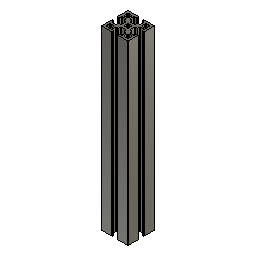
Extruder_MBXL_Cover v6 (Autodesk Fusion 360 archive; units mm, degrees)
design "MakerBeam XL"
Autodesk Fusion 360 part; units mm, degrees
sketch "Sketch1" plane through (0, 0, 0) normal (0, 0, 1) x (1, 0, 0)
  line L0 (-7.5, 7.5) -> (7.5, 7.5)
  line L1 (7.5, 7.5) -> (7.5, -7.5)
  line L2 (7.5, -7.5) -> (-7.5, -7.5)
  line L3 (-7.5, -7.5) -> (-7.5, 7.5)
  line L4 (-7.5, 7.5) -> (7.5, -7.5) construction
  line L5 (7.5, 7.5) -> (-7.5, -7.5) construction
  circle A0 centre (0, 0) radius 1.275
  line L6 (1.125, 1.125) -> (-1.125, 1.125)
  line L7 (-1.125, 1.125) -> (-1.125, -1.125)
  line L8 (-1.125, -1.125) -> (1.125, -1.125)
  line L9 (1.125, -1.125) -> (1.125, 1.125)
  line L10 (1.125, 1.125) -> (-1.125, -1.125) construction
  line L11 (-1.125, 1.125) -> (1.125, -1.125) construction
  circle A1 centre (5, 5) radius 1.275
  line L12 (6.125, 6.125) -> (3.875, 6.125)
  line L13 (3.875, 6.125) -> (3.875, 3.875)
  line L14 (3.875, 3.875) -> (6.125, 3.875)
  line L15 (6.125, 3.875) -> (6.125, 6.125)
  line L16 (6.125, 6.125) -> (3.875, 3.875) construction
  line L17 (3.875, 6.125) -> (6.125, 3.875) construction
  line L18 (7.5, 1.5) -> (2.5, 1.5)
  line L19 (2.5, 1.5) -> (2.5, -1.5)
  line L20 (2.5, -1.5) -> (7.5, -1.5)
  line L21 (7.5, -1.5) -> (7.5, 1.5)
  line L22 (7.5, 1.5) -> (2.5, -1.5) construction
  line L23 (2.5, 1.5) -> (7.5, -1.5) construction
  line L24 (6.4, 2.85) -> (3.9, 2.85)
  line L25 (3.9, 2.85) -> (3.9, -2.85)
  line L26 (3.9, -2.85) -> (6.4, -2.85)
  line L27 (6.4, -2.85) -> (6.4, 2.85)
  line L28 (6.4, 2.85) -> (3.9, -2.85) construction
  line L29 (3.9, 2.85) -> (6.4, -2.85) construction
  line L30 (-3.875, 3.875) -> (-3.875, 6.125)
  line L31 (-1.5, 7.5) -> (1.5, 2.5) construction
  line L32 (-1.5, 7.5) -> (-1.5, 2.5)
  line L33 (-6.125, 6.125) -> (-6.125, 3.875)
  line L34 (1.5, 2.5) -> (1.5, 7.5)
  line L35 (-6.125, 6.125) -> (-3.875, 3.875) construction
  circle A2 centre (-5, 5) radius 1.275
  line L36 (-1.5, 2.5) -> (1.5, 7.5) construction
  line L37 (-6.125, 3.875) -> (-3.875, 6.125) construction
  line L38 (-2.85, 6.4) -> (2.85, 3.9) construction
  line L39 (1.5, 7.5) -> (-1.5, 7.5)
  line L40 (-2.85, 3.9) -> (2.85, 3.9)
  line L41 (2.85, 3.9) -> (2.85, 6.4)
  line L42 (-6.125, 3.875) -> (-3.875, 3.875)
  line L43 (-2.85, 3.9) -> (2.85, 6.4) construction
  line L44 (-3.875, 6.125) -> (-6.125, 6.125)
  line L45 (-1.5, 2.5) -> (1.5, 2.5)
  line L46 (-2.85, 6.4) -> (-2.85, 3.9)
  line L47 (2.85, 6.4) -> (-2.85, 6.4)
  line L48 (-3.875, -3.875) -> (-6.125, -3.875)
  line L49 (-7.5, -1.5) -> (-2.5, 1.5) construction
  line L50 (-7.5, -1.5) -> (-2.5, -1.5)
  line L51 (-6.125, -6.125) -> (-3.875, -6.125)
  line L52 (-2.5, 1.5) -> (-7.5, 1.5)
  line L53 (-6.125, -6.125) -> (-3.875, -3.875) construction
  circle A3 centre (-5, -5) radius 1.275
  line L54 (-2.5, -1.5) -> (-7.5, 1.5) construction
  line L55 (-3.875, -6.125) -> (-6.125, -3.875) construction
  line L56 (-6.4, -2.85) -> (-3.9, 2.85) construction
  line L57 (-7.5, 1.5) -> (-7.5, -1.5)
  line L58 (-3.9, -2.85) -> (-3.9, 2.85)
  line L59 (-3.9, 2.85) -> (-6.4, 2.85)
  line L60 (-3.875, -6.125) -> (-3.875, -3.875)
  line L61 (-3.9, -2.85) -> (-6.4, 2.85) construction
  line L62 (-6.125, -3.875) -> (-6.125, -6.125)
  line L63 (-2.5, -1.5) -> (-2.5, 1.5)
  line L64 (-6.4, -2.85) -> (-3.9, -2.85)
  line L65 (-6.4, 2.85) -> (-6.4, -2.85)
  line L66 (3.875, -3.875) -> (3.875, -6.125)
  line L67 (1.5, -7.5) -> (-1.5, -2.5) construction
  line L68 (1.5, -7.5) -> (1.5, -2.5)
  line L69 (6.125, -6.125) -> (6.125, -3.875)
  line L70 (-1.5, -2.5) -> (-1.5, -7.5)
  line L71 (6.125, -6.125) -> (3.875, -3.875) construction
  circle A4 centre (5, -5) radius 1.275
  line L72 (1.5, -2.5) -> (-1.5, -7.5) construction
  line L73 (6.125, -3.875) -> (3.875, -6.125) construction
  line L74 (2.85, -6.4) -> (-2.85, -3.9) construction
  line L75 (-1.5, -7.5) -> (1.5, -7.5)
  line L76 (2.85, -3.9) -> (-2.85, -3.9)
  line L77 (-2.85, -3.9) -> (-2.85, -6.4)
  line L78 (6.125, -3.875) -> (3.875, -3.875)
  line L79 (2.85, -3.9) -> (-2.85, -6.4) construction
  line L80 (3.875, -6.125) -> (6.125, -6.125)
  line L81 (1.5, -2.5) -> (-1.5, -2.5)
  line L82 (2.85, -6.4) -> (2.85, -3.9)
  line L83 (-2.85, -6.4) -> (2.85, -6.4)
  point P0 (5, 5)
  point P1 (5, 0)
  point P2 (5.15, 0)
  point P3 (-5, 5)
  point P4 (0, 5)
  point P5 (0, 5.15)
  point P6 (-5, -5)
  point P7 (-5, 0)
  point P8 (-5.15, 0)
  point P9 (5, -5)
  point P10 (0, -5)
  point P11 (0, -5.15)
  dimension "d1" = 15
  dimension "d2" = 15
  dimension "d3" = 2.55
  dimension "d4" = 2.25
  dimension "d5" = 2.25
  dimension "d6" = 2.55
  dimension "d7" = 2.25
  dimension "d8" = 2.25
  dimension "d9" = 5
  dimension "d10" = 3
  dimension "d11" = 2.5
  dimension "d12" = 5.7
  dimension "d13" = 1.1
  dimension "d15" = 360
  constraint horizontal L0
  constraint perpendicular L0 L1
  constraint parallel L0 L2
  constraint parallel L1 L3
  constraint coincident L4 A0.centre
  constraint coincident L5 A0.centre
  constraint coincident A0.centre origin
  constraint horizontal L6
  constraint perpendicular L6 L7
  constraint parallel L6 L8
  constraint parallel L7 L9
  constraint coincident L10 A0.centre
  constraint coincident L11 A0.centre
  constraint coincident L5 P0
  constraint horizontal L12
  constraint perpendicular L12 L13
  constraint parallel L12 L14
  constraint parallel L13 L15
  constraint coincident L16 P0
  constraint coincident L17 P0
  constraint coincident P0 A1.centre
  constraint horizontal L18
  constraint perpendicular L18 L19
  constraint parallel L18 L20
  constraint parallel L19 L21
  constraint coincident L22 P1
  constraint coincident L23 P1
  constraint horizontal L24
  constraint perpendicular L24 L25
  constraint parallel L24 L26
  constraint parallel L25 L27
  constraint coincident L28 P2
  constraint coincident L29 P2
  measures "d1" distance of L1.end L2.end
  measures "d2" distance of L0.end L1.end
  measures "d3" diameter of A0
  measures "d4" distance of L7.end L8.end
  measures "d5" distance of L6.end L7.end
  measures "d6" diameter of A1
  measures "d7" distance of L13.end L14.end
  measures "d8" distance of L12.end L13.end
  measures "d9" distance of L19.end L20.end
  measures "d10" distance of L18.end L19.end
  measures "d11" distance of L25.end L26.end
  measures "d12" distance of L24.end L25.end
  measures "d13" distance of L1 L27
extrude "Extrude1" add sketch "Sketch1" against normal blind 100 contours L0 L1 L2 L3 L18 L19 L20 L24 L25 L26 L27 L32 L34 L40 L41 L45 L46 L47 L50 L52 L58 L59 L63 L64 L65 L68 L70 L76 L77 L81 L82 L83
fillet "Fillet1" radius 0.25 112 edges at (-7.5, 7.5, -50) (3.875, 3.875, -50) (3.875, -4.4, -50) (1.5, 3.9, -50) (1.125, 0.6, -50) (1.5, -6.4, -50) (1.5, -3.9, -50) (-3.9, 2.85, -50) (-6.125, 3.875, -50) (-6.4, 1.5, -50) (-6.125, 6.125, -50) (-2.5, 1.5, -50) (-1.5, 2.5, -50) (3.875, -6.125, -50) (-1.5, -3.9, -50) (-3.875, -4.4, -50) (6.125, -4.4, -50) (-2.85, 6.4, -50) (-6.125, -3.875, -50) (2.85, -6.4, -50) (7.5, -7.5, -50) (-2.85, 3.9, -50) (-2.5, -1.5, -50) (0.6, 1.125, -50) (6.4, 2.85, -50) (1.125, -1.125, -50) (7.5, -1.5, -50) (6.125, -6.125, -50) (-3.875, -5.6, -50) (0.6, -1.125, -50) (-6.125, 4.4, -50) (5.6, -6.125, -50) (3.9, -2.85, -50) (3.9, 1.5, -50) (5.6, 6.125, -50) (-3.9, -1.5, -50) (-3.875, 5.6, -50) (1.5, 7.5, -50) (5.6, 3.875, -50) (-5.6, 3.875, -50) (-4.4, -6.125, -50) (-0.6, -1.125, -50) (3.875, 4.4, -50) (6.125, -3.875, -50) (1.5, -2.5, -50) (6.125, 6.125, -50) (-1.5, -6.4, -50) (-6.4, -2.85, -50) (2.85, -3.9, -50) (4.4, 3.875, -50) (-4.4, 3.875, -50) (1.5, -7.5, -50) (-5.6, -3.875, -50) (-1.125, -1.125, -50) (7.5, 7.5, -50) (-3.875, 4.4, -50) (-4.4, 6.125, -50) (-6.125, -4.4, -50) (2.5, 1.5, -50) (-5.6, 6.125, -50) (6.4, 1.5, -50) (1.5, 6.4, -50) (1.125, -0.6, -50) (2.85, 3.9, -50) (-6.125, -6.125, -50) (4.4, -6.125, -50) (-1.125, -0.6, -50) (1.125, 1.125, -50) (-6.4, -1.5, -50) (-7.5, -7.5, -50) (6.125, -5.6, -50) (6.125, 3.875, -50) (-1.5, 7.5, -50) (3.875, 5.6, -50) (3.9, -1.5, -50) (-1.125, 0.6, -50) (-3.9, -2.85, -50) (-3.875, 6.125, -50) (2.85, 6.4, -50) (3.9, 2.85, -50) (-1.5, 6.4, -50) (-3.875, 3.875, -50) (3.875, -5.6, -50) (-2.85, -6.4, -50) (-1.5, 3.9, -50) (3.875, -3.875, -50) (-3.875, -6.125, -50) (-6.4, 2.85, -50) (3.875, 6.125, -50) (-5.6, -6.125, -50) (-7.5, -1.5, -50) (-3.9, 1.5, -50) (-0.6, 1.125, -50) (1.5, 2.5, -50) (6.125, 4.4, -50) (-4.4, -3.875, -50) (-1.5, -2.5, -50) (-3.875, -3.875, -50) (4.4, -3.875, -50) (5.6, -3.875, -50) (4.4, 6.125, -50) (6.4, -1.5, -50) (2.5, -1.5, -50) (-6.125, -5.6, -50) (-1.125, 1.125, -50) (-7.5, 1.5, -50) (-2.85, -3.9, -50) (7.5, 1.5, -50) (6.125, 5.6, -50) (-6.125, 5.6, -50) (-1.5, -7.5, -50) (6.4, -2.85, -50)
